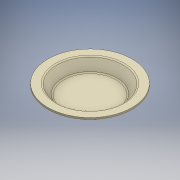
# Autodesk Inventor part: plato
Saved by Autodesk Inventor 2016 (Build 200138000, 138)
## iProperties
Created: 2016-09-16
Part Number: plato
Material: Porcelana, marfil
Document SubType Name: Modeling
Designer: Isabel
Density: 3.4 g/cm^3
Appearance: Día soleado
Author: Isabel
Autodesk Inventor part; units mm, degrees
ref_plane "YZ Plane" through (0, 0, 0) normal (1, 0, 0) x (0, 1, 0)
ref_plane "XZ Plane" through (0, 0, 0) normal (0, 1, 0) x (-1, 0, 0)
ref_plane "XY Plane" through (0, 0, 0) normal (0, 0, 1) x (1, 0, 0)
sketch "Boceto3" plane through (0, 0, 0) normal (0, 0, 1) x (1, 0, 0)
  line L0 (0, 0) -> (82.3331, 0)
  line L1 (86.4856, 2.2148) -> (103.5144, 27.6027)
  line L2 (107.6669, 29.8175) -> (125, 29.8175)
  line L3 (125, 29.8175) -> (125, 34.8175)
  line L4 (125, 34.8175) -> (102.6669, 34.8175)
  line L5 (98.5144, 32.6027) -> (81.4856, 7.2148)
  line L6 (77.3331, 5) -> (0, 5)
  line L7 (0, 5) -> (0, 0)
  arc A0 (77.3331, 5) -> (81.4856, 7.2148) centre (77.3331, 10) ccw
  arc A1 (102.6669, 34.8175) -> (98.5144, 32.6027) centre (102.6669, 29.8175) ccw
  arc A2 (107.6669, 29.8175) -> (103.5144, 27.6027) centre (107.6669, 24.8175) ccw
  arc A3 (82.3331, 0) -> (86.4856, 2.2148) centre (82.3331, 5) ccw
  point P0 (85, 0)
  point P1 (100, 34.8175)
  point P2 (80, 5)
  dimension "d6" = 125
  dimension "d8" = 80
  dimension "d9" = 5
  dimension "d10" = 5
  dimension "d12" = 100
  dimension "d13" = 85
  dimension "d16" = 5
  dimension "d17" = 5
  constraints: 16 end point, 8 point on circle, 8 tangent, 6 point on line, 4 centre point, 3 parallel, 3 perpendicular, 2 equal radius, 1 horizontal
  measures "d6" distance between parallel lines of L7 L3
  measures "d8" distance of L6.end point (80, 5)
  measures "d9" distance between parallel lines of L0 L6
  measures "d10" distance between parallel lines of L4 L2
  measures "d12" horizontal distance of L6.end point (100, 34.818)
  measures "d13" distance of L0.start point (85, 0)
  measures "d16" radius of A0
  measures "d17" radius of A1
revolve "Revolución1" add sketch "Boceto3" angle 360 about axis through (0, 5, 0) along (0, -1, 0)
move or copy body "Desplazar cuerpo1" bodies to move or copy 1 copy no rotation origin (0, 0, 0) rotation axis (1, 0, 0) rotation angle 90
move or copy body "Desplazar cuerpo2" bodies to move or copy 1 copy no translate (10, 0, 0)
